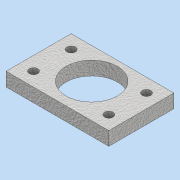
# Autodesk Inventor part: Uchwyt silnika krokowego osi X - płaski (blacha łożyska)
Saved by Autodesk Inventor 2018 (Build 220112000, 112)
## iProperties
Created: 2019-01-31
Part Number: Uchwyt silnika krokowego osi X - płaski (blacha łożyska)
Material: Ogólny
Document SubType Name: Modeling
Designer: Dawid
Density: 1 g/cm^3
Appearance: Aluminium odlewane
Author: Dawid
Autodesk Inventor part; units mm, degrees
ref_plane "YZ Plane" through (0, 0, 0) normal (1, 0, 0) x (0, 1, 0)
ref_plane "XZ Plane" through (0, 0, 0) normal (0, 1, 0) x (-1, 0, 0)
ref_plane "XY Plane" through (0, 0, 0) normal (0, 0, 1) x (1, 0, 0)
sketch "Szkic1" plane through (0, 0, 0) normal (0, 0, 1) x (1, 0, 0)
  line L0 (-30, -19) -> (30, -19)
  line L1 (30, -19) -> (30, 19)
  line L2 (30, 19) -> (-30, 19)
  line L3 (-30, 19) -> (-30, -19)
  line L4 (-30, -19) -> (30, 19) construction
  line L5 (30, -19) -> (-30, 19) construction
  line L6 (0, 19) -> (0, 1)
  circle A0 centre (0, 1) radius 15
  point P0 (0, 0)
  dimension "d0" = 60
  dimension "d1" = 38
  dimension "d2" = 18
  dimension "d3" = 30
  constraints: 14 end point, 3 midpoint, 2 parallel, 1 centre point, 1 coincident, 1 horizontal, 1 perpendicular, 1 vertical
  measures "d0" distance of L2.end L1.end
  measures "d1" distance of L1.end L0.end
  measures "d2" distance of L6.start L6.end
  measures "d3" diameter of A0
extrude "Wyciągnięcie proste1" add sketch "Szkic1" along normal blind 8
sketch "Szkic2" plane through (0, 0, 8) normal (0, 0, 1) x (1, 0, 0)
  circle A0 centre (0, 1) radius 15 projected
  line L0 (-30, -19) -> (30, -19) projected
  line L1 (30, -19) -> (30, 19) projected
  line L2 (30, 19) -> (-30, 19) projected
  line L3 (-30, 19) -> (-30, -19) projected
  line L4 (-30, 19) -> (-30, -19) projected
  line L5 (-30, 19) -> (-22, 19)
  line L6 (30, 19) -> (-30, 19) projected
  line L7 (-22, 19) -> (-22, -19)
  line L8 (30, 19) -> (22, 19)
  line L9 (22, 19) -> (22, -19)
  line L10 (-22, 19) -> (-22, 11)
  line L11 (-22, -19) -> (-22, -11)
  line L12 (22, 19) -> (22, 11)
  line L13 (22, -19) -> (22, -11)
  circle A1 centre (-22, 11) radius 2.5
  circle A2 centre (-22, -11) radius 2.5
  circle A3 centre (22, 11) radius 2.5
  circle A4 centre (22, -11) radius 2.5
  point P0 (0, 0)
  dimension "d6" = 8
  dimension "d7" = 8
  dimension "d8" = 8
  dimension "d9" = 8
  dimension "d10" = 8
  dimension "d11" = 8
  dimension "d12" = 5
  dimension "d13" = 5
  dimension "d14" = 5
  dimension "d15" = 5
  constraints: 16 end point, 8 point on line, 4 centre point, 4 coincident, 2 perpendicular
  measures "d6" distance of L2.end L5.end
  measures "d7" distance of L1.end L8.end
  measures "d8" distance of L5.end L10.end
  measures "d9" distance of L7.end L11.end
  measures "d10" distance of L8.end L12.end
  measures "d11" distance of L9.end L13.end
  measures "d12" diameter of A1
  measures "d13" diameter of A2
  measures "d14" diameter of A3
  measures "d15" diameter of A4
extrude "Wyciągnięcie proste2" cut sketch "Szkic2" against normal up to next contours A2 L7 | L7 A2 | A4 L9 | L9 A4 | A1 L7 | L7 A1 | A3 L9 | L9 A3
